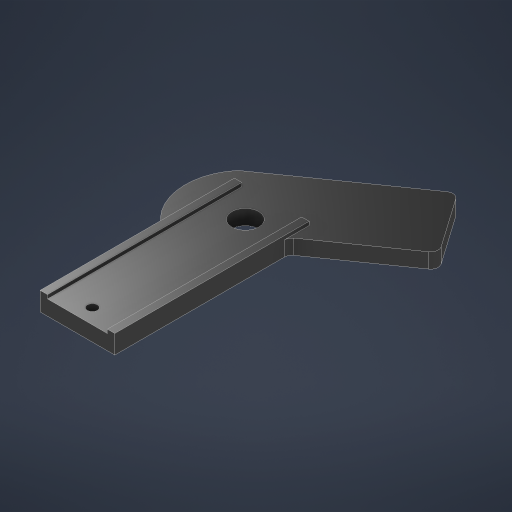
# Autodesk Inventor part: intake sleds
Saved by Autodesk Inventor 2024 (Build 280153000, 153)
## iProperties
Created: 2024-02-09
Part Number: intake sleds
Material: Generic
Document SubType Name: Modeling
Designer: elite
Density: 1 g/cm^3
Appearance: Glossy - Black
Author: elite
Autodesk Inventor part; units mm, degrees
ref_plane "YZ Plane" through (0, 0, 0) normal (1, 0, 0) x (0, 1, 0)
ref_plane "XZ Plane" through (0, 0, 0) normal (0, 1, 0) x (-1, 0, 0)
ref_plane "XY Plane" through (0, 0, 0) normal (0, 0, 1) x (1, 0, 0)
sketch "Sketch1" plane through (0, 0, 0) normal (0, 1, 0) x (-1, 0, 0)
  line L0 (0, 0) -> (31.75, 0)
  line L1 (31.75, 0) -> (31.75, -82.55)
  line L2 (31.75, -82.55) -> (0, -82.55)
  line L3 (0, -82.55) -> (0, 0)
  line L4 (31.75, -82.55) -> (28.575, -82.55)
  line L5 (0, -82.55) -> (3.175, -82.55)
  line L6 (3.175, -82.55) -> (0, -82.55)
  line L7 (0, -82.55) -> (0, 0)
  line L8 (0, 0) -> (3.175, 0)
  line L9 (3.175, 0) -> (3.175, -82.55)
  line L10 (28.575, -82.55) -> (31.75, -82.55)
  line L11 (31.75, -82.55) -> (31.75, 0)
  line L12 (31.75, 0) -> (28.575, 0)
  line L13 (28.575, 0) -> (28.575, -82.55)
  line L14 (15.875, 0) -> (15.875, -6.35)
  circle A0 centre (15.875, -6.35) radius 2.1082
  line L15 (15.875, -6.35) -> (15.875, -71.3232)
  circle A1 centre (15.875, -71.3232) radius 5.715
  dimension "d0" = 31.75
  dimension "d1" = 3.175
  dimension "d2" = 3.175
  dimension "d3" = 82.55
  dimension "d4" = 6.35
  dimension "d5" = 4.2164
  dimension "d6" = 64.9732
  dimension "d13" = 11.43
  constraints: 32 end point, 6 parallel, 3 horizontal, 3 perpendicular, 2 centre point, 2 coincident, 2 point on line, 2 vertical, 1 midpoint
  measures "d0" distance of L1.end L2.end
  measures "d1" distance of L1.end L4.end
  measures "d2" distance of L2.end L5.end
  measures "d3" distance of L8.end L5.end
  measures "d4" distance of L14.start L14.end
  measures "d5" diameter of A0
  measures "d6" distance of L15.start L15.end
  measures "d13" diameter of A1
extrude "Extrusion1" add sketch "Sketch1" along normal blind 6.35
sketch "Sketch2" plane through (0, 6.35, 0) normal (0, 1, 0) x (1, 0, 0)
  line L0 (-31.75, 0) -> (0, 0) projected
  line L1 (-31.75, 0) -> (-28.575, 0)
  line L2 (0, 0) -> (-3.175, 0)
  line L3 (0, 82.55) -> (-31.75, 82.55) projected
  line L4 (-28.575, 0) -> (-31.75, 0)
  line L5 (-31.75, 0) -> (-31.75, 82.55)
  line L6 (-31.75, 82.55) -> (-28.575, 82.55)
  line L7 (-28.575, 82.55) -> (-28.575, 0)
  line L8 (-3.175, 0) -> (0, 0)
  line L9 (0, 0) -> (0, 82.55)
  line L10 (0, 82.55) -> (-3.175, 82.55)
  line L11 (-3.175, 82.55) -> (-3.175, 0)
  dimension "d9" = 3.175
  dimension "d10" = 3.175
  constraints: 20 end point, 4 parallel, 2 horizontal, 2 perpendicular, 2 point on line
  measures "d9" distance of L0.start L1.end
  measures "d10" distance of L0.end L2.end
extrude "Extrusion2" add sketch "Sketch2" along normal blind 1.5875 contours L5 L3 L7 L0 | L11 L3 L9 L0
sketch "Sketch3" plane through (0, 0, 0) normal (0, -1, 0) x (1, 0, 0)
  line L0 (-31.75, -82.55) -> (-31.75, 0) projected
  line L1 (-31.75, -82.55) -> (-16.4111, -93.2904)
  line L2 (0, -82.55) -> (-31.75, -82.55) projected
  line L3 (-16.4111, -93.2904) -> (23.1212, -120.9712)
  line L4 (23.1212, -120.9712) -> (37.6901, -100.1648)
  line L5 (37.6901, -100.1648) -> (0, -73.7739)
  line L6 (0, 0) -> (0, -82.55) projected
  line L7 (-31.75, -82.55) -> (0, -82.55)
  dimension "d14" = 35
  dimension "d15" = 48.26
  dimension "d16" = 25.4
  constraints: 10 end point, 2 perpendicular, 1 collinear, 1 point on line
  measures "d14" angle of L2 L1
  measures "d15" distance of L1.end L3.end
  measures "d16" distance of L3.end L4.end
extrude "Extrusion3" add sketch "Sketch3" against normal blind 6.35
sketch "Sketch4" plane through (-31.75, 0, -82.55) normal (-0.5735764, 0, -0.819152) x (-0.819152, 0, 0.5735764)
  line L0 (-20.9743, 6.35) -> (-66.9854, 6.35) projected
  line L1 (0, 0) -> (0, 6.35) projected
  line L2 (-66.9854, 6.35) -> (0, 6.35)
  line L3 (0, 6.35) -> (0, 0)
  line L4 (0, 0) -> (-66.9854, 0)
  line L5 (-66.9854, 0) -> (-66.9854, 6.35)
  point P0 (21.3407, 0)
  point P1 (-20.9743, 6.35)
  constraints: 8 end point, 2 parallel, 1 horizontal, 1 perpendicular
extrude "Extrusion4" add sketch "Sketch4" along normal blind 6.35
sketch "Sketch5" plane through (0, 0, 0) normal (0, -1, 0) x (1, 0, 0)
  circle A0 centre (-15.875, -71.3232) radius 5.715 projected
  arc A1 (-31.75, -51.3533) -> (-35.3922, -87.7516) centre (-15.875, -71.3232) ccw
  line L0 (-31.75, -82.55) -> (-31.75, 0) projected
  line L1 (-31.75, -82.55) -> (-35.3922, -87.7516) projected
  line L2 (-31.75, -51.3533) -> (-31.75, -82.55)
  line L3 (-31.75, -82.55) -> (-35.3922, -87.7516)
  point P0 (0, 0)
  constraints: 4 end point, 2 point on circle, 1 centre point, 1 coincident, 1 collinear, 1 point on line, 1 vertical
extrude "Extrusion5" add sketch "Sketch5" against normal blind 6.35 contours L0 L1 A1
fillet "Fillet2" radius 3.175 3 edges at (0, 3.175, -73.7739) (19.479, 3.175, -126.1729) (37.6901, 3.175, -100.1648)
body "Solid1"
